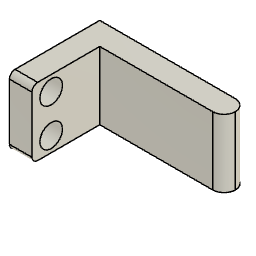
Magneto+X+trigger (Autodesk Fusion 360 design; units mm, degrees)
Autodesk Fusion 360 part; units mm, degrees
sketch "Skizze1" plane through (0, 0, 0) normal (0, 0, 1) x (1, 0, 0)
  line L0 (2, 12) -> (24, 12)
  line L1 (-2, 16) -> (24, 16)
  line L2 (24, 16) -> (24, 12)
  line L3 (2, 0) -> (2, 12)
  line L4 (-2, 0) -> (-2, 16)
  line L5 (-2, 0) -> (2, 0)
  constraint perpendicular L0 L2
  constraint perpendicular L4 L5
extrude "Extrusion1" add sketch "Skizze1" along normal blind 12
sketch "Skizze2" plane through (2, 0, 0) normal (1, 0, 0) x (0, 1, 0)
  line L0 (0, 0) -> (12, 0)
  line L1 (12, 0) -> (12, 12)
  line L2 (12, 12) -> (0, 12)
  line L3 (0, 12) -> (0, 0)
  circle A0 centre (3.4, 9.35) radius 2
  circle A1 centre (3.4, 2.65) radius 2
  dimension "d11" = 4
  dimension "d13" = 4
  measures "d11" diameter of A0
  measures "d13" diameter of A1
extrude "Extrusion2" cut sketch "Skizze2" against normal blind 12 contours A0 | A1
fillet "Abrundung1" radius 2 2 edges at (24, 16, 6) (24, 12, 6)
fillet "Abrundung2" radius 1 2 edges at (0, 0, 12) (0, 0, 0)
